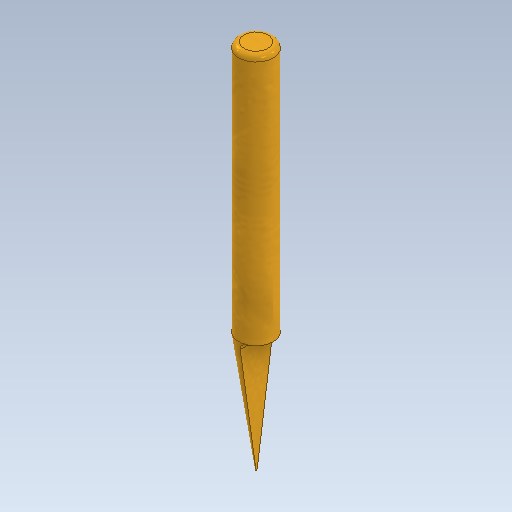
# Autodesk Inventor part: Herramienta Punta de Lanza
Saved by Autodesk Inventor 2020 (Build 240168000, 168)
## iProperties
Created: 2020-05-23
Part Number: Herramienta Punta de Lanza
Material: Generic
Document SubType Name: Modeling
Designer: Dante
Density: 1 g/cm^3
Appearance: Weld - Brass
Mass: 0.197643 g
Surface Area: 2.85715 cm^2
Volume: 0.197643 cm^3
Author: Dante
Autodesk Inventor part; units mm, degrees
ref_plane "YZ Plane" through (0, 0, 0) normal (1, 0, 0) x (0, 1, 0)
ref_plane "XZ Plane" through (0, 0, 0) normal (0, 1, 0) x (-1, 0, 0)
ref_plane "XY Plane" through (0, 0, 0) normal (0, 0, 1) x (1, 0, 0)
sketch "Sketch1" plane through (0, 0, 0) normal (0, 0, 1) x (1, 0, 0)
  line L0 (0, 23) -> (-1.087, 23)
  line L1 (-1.587, 22.5) -> (-1.587, 0)
  line L2 (0, 23) -> (0, -11)
  line L3 (0, -11) -> (0, -10.95)
  line L4 (0, -11) -> (-0.05, -11)
  line L5 (-0.05, -11) -> (-1.587, 0)
  arc A0 (-1.087, 23) -> (-1.587, 22.5) centre (-1.087, 22.5) ccw
  point P0 (-1.587, 23)
  dimension "d1" = 1.587
  dimension "d8" = 0.05
  dimension "d13" = 0.5
  constraints: 12 end point, 3 point on line, 2 point on circle, 2 tangent, 1 centre point, 1 horizontal, 1 vertical
  measures "d1" distance of L0.start point (-1.587, 23)
  measures "d8" distance of L2.end L4.end
  measures "d13" radius of A0
revolve "Revolution1" add sketch "Sketch1" angle 360 about axis through (0, 23, 0) along (0, -1, 0)
sketch "Sketch2" plane through (0, -11, 0) normal (0, -1, 0) x (1, 0, 0)
  line L0 (0.05, 1.7032) -> (0.05, -1.887)
  line L1 (0.05, -1.887) -> (1.6041, -1.887)
  line L2 (1.6041, -1.887) -> (1.6041, 1.7032)
  line L3 (1.6041, 1.7032) -> (0.05, 1.7032)
  point P0 (0, 0)
  dimension "d10" = 0.05
  constraints: 8 end point, 3 perpendicular, 1 vertical
  measures "d10" distance from line of point (0, 0) L0
extrude "Extrusion1" cut sketch "Sketch2" against normal blind 11
fillet "Fillet1" radius 0.65 1 edges at (0.05, 0, 0)
body "Solid1"
